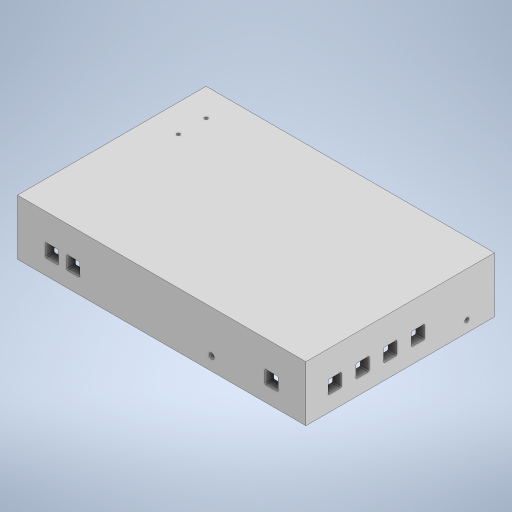
# Autodesk Inventor part: TouchShakerBox
Saved by Autodesk Inventor 2023 (Build 270158000, 158)
## iProperties
Created: 2023-03-28
Part Number: TouchShakerBox
Material: Generic
Document SubType Name: Modeling
Designer: yousefi
Density: 1 g/cm^3
Appearance: Default
Author: yousefi
Autodesk Inventor part; units mm, degrees
ref_plane "YZ Plane" through (0, 0, 0) normal (1, 0, 0) x (0, 1, 0)
ref_plane "XZ Plane" through (0, 0, 0) normal (0, 1, 0) x (-1, 0, 0)
ref_plane "XY Plane" through (0, 0, 0) normal (0, 0, 1) x (1, 0, 0)
sketch "Sketch1" plane through (0, 0, 0) normal (0, 1, 0) x (-1, 0, 0)
  line L0 (0, -170) -> (260, -170)
  line L1 (260, -170) -> (260, 0)
  line L2 (260, 0) -> (0, 0)
  line L3 (0, 0) -> (0, -170)
  dimension "d2" = 260
  dimension "d3" = 170
  constraints: 8 end point, 2 parallel, 1 coincident, 1 horizontal, 1 perpendicular
  measures "d2" distance of L2.end L1.end
  measures "d3" distance of L1.end L0.end
extrude "Box" add sketch "Sketch1" along normal blind 50
sketch "Sketch2" plane through (0, 0, 0) normal (1, 0, 0) x (0, 0, -1)
  line L0 (31, 14) -> (21, 14)
  line L1 (20, 15) -> (20, 25)
  line L2 (21, 26) -> (31, 26)
  line L3 (32, 25) -> (32, 15)
  arc A0 (21, 26) -> (20, 25) centre (21, 25) ccw
  arc A1 (32, 25) -> (31, 26) centre (31, 25) ccw
  arc A2 (31, 14) -> (32, 15) centre (31, 15) ccw
  arc A3 (20, 15) -> (21, 14) centre (21, 15) ccw
  line L4 (56, 14) -> (46, 14)
  line L5 (45, 15) -> (45, 25)
  line L6 (46, 26) -> (56, 26)
  line L7 (57, 25) -> (57, 15)
  arc A4 (46, 26) -> (45, 25) centre (46, 25) ccw
  arc A5 (57, 25) -> (56, 26) centre (56, 25) ccw
  arc A6 (56, 14) -> (57, 15) centre (56, 15) ccw
  arc A7 (45, 15) -> (46, 14) centre (46, 15) ccw
  line L8 (81, 14) -> (71, 14)
  line L9 (70, 15) -> (70, 25)
  line L10 (71, 26) -> (81, 26)
  line L11 (82, 25) -> (82, 15)
  arc A8 (71, 26) -> (70, 25) centre (71, 25) ccw
  arc A9 (82, 25) -> (81, 26) centre (81, 25) ccw
  arc A10 (81, 14) -> (82, 15) centre (81, 15) ccw
  arc A11 (70, 15) -> (71, 14) centre (71, 15) ccw
  line L12 (106, 14) -> (96, 14)
  line L13 (95, 15) -> (95, 25)
  line L14 (96, 26) -> (106, 26)
  line L15 (107, 25) -> (107, 15)
  arc A12 (96, 26) -> (95, 25) centre (96, 25) ccw
  arc A13 (107, 25) -> (106, 26) centre (106, 25) ccw
  arc A14 (106, 14) -> (107, 15) centre (106, 15) ccw
  arc A15 (95, 15) -> (96, 14) centre (96, 15) ccw
  line L16 (0, 0) -> (0, 50) construction
  line L17 (0, 0) -> (170, 0) construction
  point P0 (32, 14)
  point P1 (20, 26)
  point P2 (20, 14)
  point P3 (32, 26)
  point P4 (57, 14)
  point P5 (45, 26)
  point P6 (45, 14)
  point P7 (57, 26)
  point P8 (82, 14)
  point P9 (70, 26)
  point P10 (70, 14)
  point P11 (82, 26)
  point P12 (107, 14)
  point P13 (95, 26)
  point P14 (95, 14)
  point P15 (107, 26)
  point P16 (20, 20)
  dimension "d6" = 12
  dimension "d7" = 12
  dimension "d72" = 1
  dimension "d73" = 12
  dimension "d74" = 12
  dimension "d75" = 1
  dimension "d76" = 12
  dimension "d77" = 12
  dimension "d78" = 1
  dimension "d79" = 12
  dimension "d80" = 12
  dimension "d81" = 1
  dimension "d82" = 14
  dimension "d83" = 20
  dimension "d84" = 25
  dimension "d87" = 25
  dimension "d88" = 25
  constraints: 32 end point, 32 point on circle, 32 point on line, 32 tangent, 16 centre point, 12 equal radius, 8 parallel, 4 horizontal, 4 perpendicular, 3 collinear, 1 midpoint
  measures "d6" distance of point (20, 26) point (32, 26)
  measures "d7" distance of point (20, 14) point (20, 26)
  measures "d72" radius of A0
  measures "d73" distance of point (45, 26) point (57, 26)
  measures "d74" distance of point (45, 14) point (45, 26)
  measures "d75" radius of A4
  measures "d76" distance of point (70, 26) point (82, 26)
  measures "d77" distance of point (70, 14) point (70, 26)
  measures "d78" radius of A8
  measures "d79" distance of point (95, 26) point (107, 26)
  measures "d80" distance of point (95, 14) point (95, 26)
  measures "d81" radius of A12
  measures "d82" distance between parallel lines of L17 L0
  measures "d83" distance between parallel lines of L16 L1
  measures "d84" distance from line of point (20, 20) L5
  measures "d87" distance between parallel lines of L9 L5
  measures "d88" distance between parallel lines of L13 L9
extrude "Ethernet" cut sketch "Sketch2" against normal blind 20
sketch "Sketch6" plane through (-260, 0, 0) normal (0, 0, 1) x (1, 0, 0)
  line L0 (36, 26) -> (26, 26)
  line L1 (25, 25) -> (25, 15)
  line L2 (26, 14) -> (36, 14)
  line L3 (37, 15) -> (37, 25)
  line L4 (0, 0) -> (0, 50) projected
  line L5 (0, 0) -> (260, 0) projected
  arc A0 (26, 26) -> (25, 25) centre (26, 25) ccw
  arc A1 (37, 25) -> (36, 26) centre (36, 25) ccw
  arc A2 (36, 14) -> (37, 15) centre (36, 15) ccw
  arc A3 (25, 15) -> (26, 14) centre (26, 15) ccw
  line L6 (55.35, 26) -> (45.35, 26)
  line L7 (44.35, 25) -> (44.35, 15)
  line L8 (45.35, 14) -> (55.35, 14)
  line L9 (56.35, 15) -> (56.35, 25)
  arc A4 (45.35, 26) -> (44.35, 25) centre (45.35, 25) ccw
  arc A5 (56.35, 25) -> (55.35, 26) centre (55.35, 25) ccw
  arc A6 (55.35, 14) -> (56.35, 15) centre (55.35, 15) ccw
  arc A7 (44.35, 15) -> (45.35, 14) centre (45.35, 15) ccw
  point P0 (37, 26)
  point P1 (25, 14)
  point P2 (25, 26)
  point P3 (37, 14)
  point P4 (56.35, 26)
  point P5 (44.35, 14)
  point P6 (44.35, 26)
  point P7 (56.35, 14)
  dimension "d22" = 12
  dimension "d23" = 12
  dimension "d92" = 25
  dimension "d93" = 14
  dimension "d94" = 1
  dimension "d95" = 12
  dimension "d96" = 12
  dimension "d97" = 1
  dimension "d99" = 7.35
  constraints: 16 end point, 16 point on circle, 16 point on line, 16 tangent, 8 centre point, 6 equal radius, 4 parallel, 2 horizontal, 2 perpendicular, 1 collinear
  measures "d22" distance of point (37, 14) point (25, 14)
  measures "d23" distance of point (25, 14) point (25, 26)
  measures "d92" distance between parallel lines of L4 L1
  measures "d93" distance between parallel lines of L5 L2
  measures "d94" radius of A0
  measures "d95" distance of point (56.35, 14) point (44.35, 14)
  measures "d96" distance of point (44.35, 14) point (44.35, 26)
  measures "d97" radius of A4
  measures "d99" distance between parallel lines of L7 L3
extrude "Rotary-Ethernet" cut sketch "Sketch6" against normal blind 20
sketch "Sketch9" plane through (0, 50, 0) normal (0, 1, 0) x (1, 0, 0)
  circle A0 centre (-235, 120) radius 1.5
  line L0 (-260, 170) -> (-260, 0) construction
  line L1 (0, 170) -> (-260, 170) construction
  circle A1 centre (-235, 145) radius 1.5
  point P0 (0, 0)
  dimension "d33" = 3
  dimension "d68" = 25
  dimension "d69" = 50
  dimension "d70" = 25
  dimension "d71" = 25
  constraints: 2 centre point, 1 equal radius
  measures "d33" diameter of A0
  measures "d68" distance from line of L0 A0.centre
  measures "d69" distance from line of L1 A0.centre
  measures "d70" distance from line of L1 A1.centre
  measures "d71" distance from line of L0 A1.centre
extrude "Spout1" cut sketch "Sketch9" against normal blind 20
sketch "Sketch11" plane through (0, 0, -170) normal (0, 0, -1) x (-1, 0, 0)
  line L0 (136, 14) -> (128, 14)
  line L1 (127, 15) -> (127, 23)
  line L2 (128, 24) -> (136, 24)
  line L3 (137, 23) -> (137, 15)
  line L4 (0, 0) -> (260, 0) projected
  line L5 (0, 0) -> (0, 50) projected
  arc A0 (128, 24) -> (127, 23) centre (128, 23) ccw
  arc A1 (137, 23) -> (136, 24) centre (136, 23) ccw
  arc A2 (136, 14) -> (137, 15) centre (136, 15) ccw
  arc A3 (127, 15) -> (128, 14) centre (128, 15) ccw
  point P0 (0, 0)
  point P1 (137, 14)
  point P2 (127, 24)
  point P3 (127, 14)
  point P4 (137, 24)
  dimension "d39" = 10
  dimension "d40" = 10
  dimension "d105" = 14
  dimension "d106" = 127
  dimension "d107" = 1
  constraints: 8 end point, 8 point on circle, 8 point on line, 8 tangent, 4 centre point, 3 equal radius, 2 parallel, 1 horizontal, 1 perpendicular
  measures "d39" distance of point (127, 24) point (137, 24)
  measures "d40" distance of point (127, 14) point (127, 24)
  measures "d105" distance between parallel lines of L4 L0
  measures "d106" distance between parallel lines of L5 L1
  measures "d107" radius of A0
extrude "Teensy usb" cut sketch "Sketch11" against normal blind 10
sketch "Sketch13" plane through (-260, 0, 0) normal (0, 0, 1) x (1, 0, 0)
  line L0 (224, 26) -> (234, 26)
  line L1 (235, 25) -> (235, 15)
  line L2 (234, 14) -> (224, 14)
  line L3 (223, 15) -> (223, 25)
  line L4 (260, 0) -> (260, 50) projected
  line L5 (0, 0) -> (260, 0) projected
  arc A0 (224, 26) -> (223, 25) centre (224, 25) ccw
  arc A1 (235, 25) -> (234, 26) centre (234, 25) ccw
  arc A2 (234, 14) -> (235, 15) centre (234, 15) ccw
  arc A3 (223, 15) -> (224, 14) centre (224, 15) ccw
  point P0 (223, 26)
  point P1 (235, 14)
  point P2 (235, 26)
  point P3 (223, 14)
  dimension "d43" = 12
  dimension "d44" = 12
  dimension "d89" = 25
  dimension "d90" = 14
  dimension "d91" = 1
  constraints: 8 end point, 8 point on circle, 8 point on line, 8 tangent, 4 centre point, 3 equal radius, 2 parallel, 1 horizontal, 1 perpendicular
  measures "d43" distance of point (235, 14) point (223, 14)
  measures "d44" distance of point (235, 26) point (235, 14)
  measures "d89" distance between parallel lines of L4 L1
  measures "d90" distance between parallel lines of L5 L2
  measures "d91" radius of A0
extrude "Teensy shield" cut sketch "Sketch13" against normal blind 10
sketch "power 5 v" plane through (0, 0, -170) normal (0, 0, -1) x (-1, 0, 0)
  circle A0 centre (118, 11) radius 2
  line L0 (0, 0) -> (260, 0) projected
  line L1 (136, 14) -> (128, 14) projected
  point P0 (132, 14)
  dimension "d47" = 4
  dimension "d108" = 11
  dimension "d109" = 14
  constraints: 1 centre point, 1 midpoint
  measures "d47" diameter of A0
  measures "d108" distance from line of L0 A0.centre
  measures "d109" horizontal distance of point (132, 14) A0.centre
extrude "Power5" cut sketch "power 5 v" against normal blind 20
sketch "power9" plane through (0, 0, 0) normal (1, 0, 0) x (0, 0, -1)
  circle A0 centre (145, 10) radius 2
  line L0 (0, 0) -> (170, 0) projected
  line L1 (170, 0) -> (170, 50) projected
  dimension "d50" = 4
  dimension "d85" = 10
  dimension "d86" = 25
  constraints: 1 centre point
  measures "d50" diameter of A0
  measures "d85" distance from line of L0 A0.centre
  measures "d86" distance from line of L1 A0.centre
extrude "Power 9" cut sketch "power9" against normal blind 20
sketch "Power121" plane through (-260, 0, 0) normal (0, 0, 1) x (1, 0, 0)
  circle A0 centre (175, 12) radius 2.5
  line L0 (0, 0) -> (260, 0) projected
  arc A1 (234, 14) -> (235, 15) centre (234, 15) ccw projected
  line L1 (234, 14) -> (224, 14) projected
  arc A2 (223, 15) -> (224, 14) centre (224, 15) ccw projected
  line L2 (223, 15) -> (223, 25) projected
  arc A3 (224, 26) -> (223, 25) centre (224, 25) ccw projected
  line L3 (224, 26) -> (234, 26) projected
  arc A4 (235, 25) -> (234, 26) centre (234, 25) ccw projected
  line L4 (235, 25) -> (235, 15) projected
  line L5 (25, 15) -> (25, 25) projected
  arc A5 (26, 26) -> (25, 25) centre (26, 25) ccw projected
  line L6 (26, 26) -> (36, 26) projected
  arc A6 (37, 25) -> (36, 26) centre (36, 25) ccw projected
  line L7 (37, 25) -> (37, 15) projected
  arc A7 (36, 14) -> (37, 15) centre (36, 15) ccw projected
  line L8 (36, 14) -> (26, 14) projected
  arc A8 (25, 15) -> (26, 14) centre (26, 15) ccw projected
  arc A9 (45.35, 26) -> (44.35, 25) centre (45.35, 25) ccw projected
  line L9 (45.35, 26) -> (55.35, 26) projected
  arc A10 (56.35, 25) -> (55.35, 26) centre (55.35, 25) ccw projected
  line L10 (56.35, 25) -> (56.35, 15) projected
  arc A11 (55.35, 14) -> (56.35, 15) centre (55.35, 15) ccw projected
  line L11 (55.35, 14) -> (45.35, 14) projected
  arc A12 (44.35, 15) -> (45.35, 14) centre (45.35, 15) ccw projected
  line L12 (44.35, 15) -> (44.35, 25) projected
  line L13 (0, 0) -> (260, 0) projected
  line L14 (260, 0) -> (260, 50) projected
  line L15 (0, 50) -> (260, 50) projected
  line L16 (0, 0) -> (0, 50) projected
  dimension "d53" = 5
  dimension "d100" = 12
  dimension "d101" = 85
  constraints: 1 centre point
  measures "d53" diameter of A0
  measures "d100" distance from line of L0 A0.centre
  measures "d101" distance from line of L14 A0.centre
extrude "Power12" cut sketch "Power121" against normal blind 20 contours A0
sketch "Rotary USB1" plane through (-260, 0, -170) normal (-1, 0, 0) x (0, 0, 1)
  line L0 (137, 24) -> (129, 24)
  line L1 (128, 23) -> (128, 15)
  line L2 (129, 14) -> (137, 14)
  line L3 (138, 15) -> (138, 23)
  line L4 (0, 0) -> (170, 0) projected
  line L5 (170, 0) -> (170, 50) projected
  arc A0 (138, 23) -> (137, 24) centre (137, 23) ccw
  arc A1 (137, 14) -> (138, 15) centre (137, 15) ccw
  arc A2 (128, 15) -> (129, 14) centre (129, 15) ccw
  arc A3 (129, 24) -> (128, 23) centre (129, 23) ccw
  point P0 (170, 0)
  point P1 (138, 24)
  point P2 (128, 14)
  point P3 (128, 24)
  point P4 (138, 14)
  dimension "d58" = 10
  dimension "d59" = 10
  dimension "d102" = 14
  dimension "d103" = 32
  dimension "d104" = 1
  constraints: 8 end point, 8 point on circle, 8 point on line, 8 tangent, 4 centre point, 3 equal radius, 2 parallel, 1 horizontal, 1 perpendicular
  measures "d58" distance of point (138, 14) point (128, 14)
  measures "d59" distance of point (128, 14) point (128, 24)
  measures "d102" distance between parallel lines of L4 L2
  measures "d103" distance between parallel lines of L5 L3
  measures "d104" radius of A0
extrude "Rotary USB" cut sketch "Rotary USB1" against normal blind 20
sketch "Sketch19" plane through (0, 0, 0) normal (0, -1, 0) x (1, 0, 0)
  line L0 (-260, -170) -> (-260, 0) construction
  line L1 (0, -170) -> (-260, -170) construction
  line L2 (0, 0) -> (0, -170) construction
  line L3 (-260, 0) -> (0, 0) construction
  line L4 (-8, -162) -> (-252, -162)
  line L5 (-252, -162) -> (-252, -8)
  line L6 (-252, -8) -> (-8, -8)
  line L7 (-8, -8) -> (-8, -162)
  dimension "d62" = 8
  dimension "d63" = 8
  dimension "d64" = 8
  dimension "d65" = 8
  constraints: 8 end point, 2 parallel, 1 horizontal, 1 perpendicular
  measures "d62" distance between parallel lines of L1 L4
  measures "d63" distance between parallel lines of L3 L6
  measures "d64" distance between parallel lines of L2 L7
  measures "d65" distance between parallel lines of L0 L5
extrude "Extrusion17" cut sketch "Sketch19" against normal blind 46
body "Solid1"
